Autodesk Fusion 360 part; units mm, degrees
(part 6 of 8)
equation "d149 = FootHeight"
equation "d151 = ( BaseX + TowerFrame + TowerClearance ) + ( ( ( TowerWidth - 2 * ( TowerFrame + TowerClearance ) ) - 11 mm ) - PegSize / 2 - FitClearance )"
equation "d152 = ( BaseY ) + ( ( 11 mm ) - PegSize / 2 - FitClearance )"
equation "d153 = PegSize + 2 * FitClearance"
equation "d154 = PegSize + 2 * FitClearance"
equation "d155 = PegHeight + 0.3 mm"
equation "d157 = FootHeight"
equation "d159 = ( BaseX + TowerFrame + TowerClearance ) + ( ( ( TowerWidth - 2 * ( TowerFrame + TowerClearance ) ) - 11 mm ) - PegSize / 2 - FitClearance )"
equation "d160 = ( BaseY ) + ( ( ( Depth ) - 11 mm ) - PegSize / 2 - FitClearance )"
equation "d161 = PegSize + 2 * FitClearance"
equation "d162 = PegSize + 2 * FitClearance"
equation "d163 = PegHeight + 0.3 mm"
equation "d165 = ( FootHeight ) + PanHeight - DeckThick"
equation "d167 = ( BaseX + TowerFrame + TowerClearance ) + ( Wall + DeckClearance )"
equation "d168 = ( BaseY ) + ( Wall + DeckClearance )"
equation "d169 = ( TowerWidth - 2 * ( TowerFrame + TowerClearance ) ) - 2 * ( Wall + DeckClearance )"
equation "d170 = ( Depth ) - 2 * ( Wall + DeckClearance )"
equation "d171 = DeckThick"
equation "d173 = ( FootHeight ) + PanHeight - DeckThick"
equation "d175 = ( BaseX + TowerFrame + TowerClearance ) + ( ( ( ( TowerWidth - 2 * ( TowerFrame + TowerClearance ) ) - ( 12 * SlotPitch + SlotWidth ) ) / 2 ) + ( 0 * SlotPitch ) )"
equation "d176 = ( BaseY ) + ( Wall + DeckClearance + RimBorder )"
equation "d177 = SlotWidth"
equation "d178 = ( Depth ) - 2 * ( Wall + DeckClearance + RimBorder )"
equation "d179 = DeckThick"
equation "d181 = ( FootHeight ) + PanHeight - DeckThick"
equation "d183 = ( BaseX + TowerFrame + TowerClearance ) + ( ( ( ( TowerWidth - 2 * ( TowerFrame + TowerClearance ) ) - ( 12 * SlotPitch + SlotWidth ) ) / 2 ) + ( 1 * SlotPitch ) )"
equation "d184 = ( BaseY ) + ( Wall + DeckClearance + RimBorder )"
equation "d185 = SlotWidth"
equation "d186 = ( Depth ) - 2 * ( Wall + DeckClearance + RimBorder )"
equation "d187 = DeckThick"
equation "d189 = ( FootHeight ) + PanHeight - DeckThick"
equation "d191 = ( BaseX + TowerFrame + TowerClearance ) + ( ( ( ( TowerWidth - 2 * ( TowerFrame + TowerClearance ) ) - ( 12 * SlotPitch + SlotWidth ) ) / 2 ) + ( 2 * SlotPitch ) )"
equation "d192 = ( BaseY ) + ( Wall + DeckClearance + RimBorder )"
equation "d193 = SlotWidth"
equation "d194 = ( Depth ) - 2 * ( Wall + DeckClearance + RimBorder )"
equation "d195 = DeckThick"
equation "d197 = ( FootHeight ) + PanHeight - DeckThick"
equation "d199 = ( BaseX + TowerFrame + TowerClearance ) + ( ( ( ( TowerWidth - 2 * ( TowerFrame + TowerClearance ) ) - ( 12 * SlotPitch + SlotWidth ) ) / 2 ) + ( 3 * SlotPitch ) )"
equation "d200 = ( BaseY ) + ( Wall + DeckClearance + RimBorder )"
equation "d201 = SlotWidth"
equation "d202 = ( Depth ) - 2 * ( Wall + DeckClearance + RimBorder )"
equation "d203 = DeckThick"
equation "d205 = ( FootHeight ) + PanHeight - DeckThick"
equation "d207 = ( BaseX + TowerFrame + TowerClearance ) + ( ( ( ( TowerWidth - 2 * ( TowerFrame + TowerClearance ) ) - ( 12 * SlotPitch + SlotWidth ) ) / 2 ) + ( 4 * SlotPitch ) )"
equation "d208 = ( BaseY ) + ( Wall + DeckClearance + RimBorder )"
equation "d209 = SlotWidth"
equation "d210 = ( Depth ) - 2 * ( Wall + DeckClearance + RimBorder )"
equation "d211 = DeckThick"
equation "d213 = ( FootHeight ) + PanHeight - DeckThick"
equation "d215 = ( BaseX + TowerFrame + TowerClearance ) + ( ( ( ( TowerWidth - 2 * ( TowerFrame + TowerClearance ) ) - ( 12 * SlotPitch + SlotWidth ) ) / 2 ) + ( 5 * SlotPitch ) )"
equation "d216 = ( BaseY ) + ( Wall + DeckClearance + RimBorder )"
equation "d217 = SlotWidth"
equation "d218 = ( Depth ) - 2 * ( Wall + DeckClearance + RimBorder )"
equation "d219 = DeckThick"
equation "d221 = ( FootHeight ) + PanHeight - DeckThick"
equation "d223 = ( BaseX + TowerFrame + TowerClearance ) + ( ( ( ( TowerWidth - 2 * ( TowerFrame + TowerClearance ) ) - ( 12 * SlotPitch + SlotWidth ) ) / 2 ) + ( 6 * SlotPitch ) )"
equation "d224 = ( BaseY ) + ( Wall + DeckClearance + RimBorder )"
equation "d225 = SlotWidth"
equation "d226 = ( Depth ) - 2 * ( Wall + DeckClearance + RimBorder )"
equation "d227 = DeckThick"
equation "d229 = ( FootHeight ) + PanHeight - DeckThick"
equation "d231 = ( BaseX + TowerFrame + TowerClearance ) + ( ( ( ( TowerWidth - 2 * ( TowerFrame + TowerClearance ) ) - ( 12 * SlotPitch + SlotWidth ) ) / 2 ) + ( 7 * SlotPitch ) )"
equation "d232 = ( BaseY ) + ( Wall + DeckClearance + RimBorder )"
equation "d233 = SlotWidth"
equation "d234 = ( Depth ) - 2 * ( Wall + DeckClearance + RimBorder )"
equation "d235 = DeckThick"
equation "d237 = ( FootHeight ) + PanHeight - DeckThick"
equation "d239 = ( BaseX + TowerFrame + TowerClearance ) + ( ( ( ( TowerWidth - 2 * ( TowerFrame + TowerClearance ) ) - ( 12 * SlotPitch + SlotWidth ) ) / 2 ) + ( 8 * SlotPitch ) )"
equation "d240 = ( BaseY ) + ( Wall + DeckClearance + RimBorder )"
equation "d241 = SlotWidth"
equation "d242 = ( Depth ) - 2 * ( Wall + DeckClearance + RimBorder )"
equation "d243 = DeckThick"
equation "d245 = ( FootHeight ) + PanHeight - DeckThick"
equation "d247 = ( BaseX + TowerFrame + TowerClearance ) + ( ( ( ( TowerWidth - 2 * ( TowerFrame + TowerClearance ) ) - ( 12 * SlotPitch + SlotWidth ) ) / 2 ) + ( 9 * SlotPitch ) )"
equation "d248 = ( BaseY ) + ( Wall + DeckClearance + RimBorder )"
equation "d249 = SlotWidth"
equation "d250 = ( Depth ) - 2 * ( Wall + DeckClearance + RimBorder )"
equation "d251 = DeckThick"
equation "d253 = ( FootHeight ) + PanHeight - DeckThick"
equation "d255 = ( BaseX + TowerFrame + TowerClearance ) + ( ( ( ( TowerWidth - 2 * ( TowerFrame + TowerClearance ) ) - ( 12 * SlotPitch + SlotWidth ) ) / 2 ) + ( 10 * SlotPitch ) )"
equation "d256 = ( BaseY ) + ( Wall + DeckClearance + RimBorder )"
equation "d257 = SlotWidth"
equation "d258 = ( Depth ) - 2 * ( Wall + DeckClearance + RimBorder )"
equation "d259 = DeckThick"
equation "d261 = ( FootHeight ) + PanHeight - DeckThick"
equation "d263 = ( BaseX + TowerFrame + TowerClearance ) + ( ( ( ( TowerWidth - 2 * ( TowerFrame + TowerClearance ) ) - ( 12 * SlotPitch + SlotWidth ) ) / 2 ) + ( 11 * SlotPitch ) )"
equation "d264 = ( BaseY ) + ( Wall + DeckClearance + RimBorder )"
equation "d265 = SlotWidth"
equation "d266 = ( Depth ) - 2 * ( Wall + DeckClearance + RimBorder )"
equation "d267 = DeckThick"
equation "d269 = ( FootHeight ) + PanHeight - DeckThick"
equation "d271 = ( BaseX + TowerFrame + TowerClearance ) + ( ( ( ( TowerWidth - 2 * ( TowerFrame + TowerClearance ) ) - ( 12 * SlotPitch + SlotWidth ) ) / 2 ) + ( 12 * SlotPitch ) )"
equation "d272 = ( BaseY ) + ( Wall + DeckClearance + RimBorder )"
equation "d273 = SlotWidth"
equation "d274 = ( Depth ) - 2 * ( Wall + DeckClearance + RimBorder )"
equation "d275 = DeckThick"
equation "d277 = ( FootHeight ) + PanHeight - DeckThick"
equation "d279 = ( BaseX + TowerFrame + TowerClearance ) + ( ( TowerWidth - 2 * ( TowerFrame + TowerClearance ) ) / 2 - 8 mm )"
equation "d280 = ( BaseY ) + ( ( Depth ) - Wall - DeckClearance - 4 mm )"
equation "d283 = DeckThick"
equation "d287 = ( BaseX + TowerFrame + TowerClearance ) + ( ( 11 mm ) - FootSize / 2 )"
equation "d288 = ( BaseY ) + ( ( 11 mm ) - FootSize / 2 )"
equation "d289 = FootSize"
equation "d290 = FootSize"
equation "d291 = FootHeight"
equation "d293 = FootHeight"
equation "d295 = ( BaseX + TowerFrame + TowerClearance ) + ( ( 11 mm ) - PegSize / 2 )"
equation "d296 = ( BaseY ) + ( ( 11 mm ) - PegSize / 2 )"
equation "d297 = PegSize"
equation "d298 = PegSize"
equation "d299 = PegHeight"
equation "d303 = ( BaseX + TowerFrame + TowerClearance ) + ( ( 11 mm ) - FootSize / 2 )"
equation "d304 = ( BaseY ) + ( ( ( Depth ) - 11 mm ) - FootSize / 2 )"
equation "d305 = FootSize"
equation "d306 = FootSize"
equation "d307 = FootHeight"
equation "d309 = FootHeight"
equation "d311 = ( BaseX + TowerFrame + TowerClearance ) + ( ( 11 mm ) - PegSize / 2 )"
equation "d312 = ( BaseY ) + ( ( ( Depth ) - 11 mm ) - PegSize / 2 )"
equation "d313 = PegSize"
equation "d314 = PegSize"
equation "d315 = PegHeight"
equation "d319 = ( BaseX + TowerFrame + TowerClearance ) + ( ( ( TowerWidth - 2 * ( TowerFrame + TowerClearance ) ) - 11 mm ) - FootSize / 2 )"
equation "d320 = ( BaseY ) + ( ( 11 mm ) - FootSize / 2 )"
equation "d321 = FootSize"
equation "d322 = FootSize"
equation "d323 = FootHeight"
equation "d325 = FootHeight"
equation "d327 = ( BaseX + TowerFrame + TowerClearance ) + ( ( ( TowerWidth - 2 * ( TowerFrame + TowerClearance ) ) - 11 mm ) - PegSize / 2 )"
equation "d328 = ( BaseY ) + ( ( 11 mm ) - PegSize / 2 )"
equation "d329 = PegSize"
equation "d330 = PegSize"
equation "d331 = PegHeight"
equation "d335 = ( BaseX + TowerFrame + TowerClearance ) + ( ( ( TowerWidth - 2 * ( TowerFrame + TowerClearance ) ) - 11 mm ) - FootSize / 2 )"
equation "d336 = ( BaseY ) + ( ( ( Depth ) - 11 mm ) - FootSize / 2 )"
equation "d337 = FootSize"
equation "d338 = FootSize"
equation "d339 = FootHeight"
equation "d341 = FootHeight"
equation "d343 = ( BaseX + TowerFrame + TowerClearance ) + ( ( ( TowerWidth - 2 * ( TowerFrame + TowerClearance ) ) - 11 mm ) - PegSize / 2 )"
equation "d344 = ( BaseY ) + ( ( ( Depth ) - 11 mm ) - PegSize / 2 )"
equation "d345 = PegSize"
equation "d346 = PegSize"
equation "d347 = PegHeight"
equation "d349 = FootHeight"
equation "d351 = ( BaseX + TowerWidth + ModuleGap ) + ( 0 mm )"
equation "d352 = ( BaseY ) + ( 0 mm )"
equation "d353 = LeftRun - TowerWidth - ModuleGap"
equation "d354 = Depth"
equation "d355 = PanHeight"
equation "d359 = ( BaseX + TowerWidth + ModuleGap ) + ( Wall )"
equation "d361 = -( -( ( FootHeight ) + FloorMin + DrainExtension * tan(DrainSlope) + ( ( Depth ) - ( Wall ) ) * tan(DrainSlope) ) )"
equation "d362 = ( ( BaseY ) + ( Wall ) )"
equation "d363 = -( -( ( FootHeight ) + FloorMin + DrainExtension * tan(DrainSlope) + ( ( Depth ) - ( ( Depth ) - Wall ) ) * tan(DrainSlope) ) )"
equation "d364 = ( ( BaseY ) + ( ( Depth ) - Wall ) )"
equation "d365 = -( -( ( FootHeight ) + PanHeight + 1 mm ) )"
equation "d366 = ( LeftRun - TowerWidth - ModuleGap ) - 2 * Wall"
equation "d368 = ( BaseX + TowerWidth + ModuleGap ) + ( ( ( LeftRun - TowerWidth - ModuleGap ) / 2 ) - DrainWidth / 2 - Wall )"
equation "d370 = -( -( FootHeight ) )"
equation "d371 = ( ( BaseY ) + ( ( Depth ) - Wall ) )"
equation "d372 = ( ( BaseY ) + ( ( Depth ) + DrainExtension ) )"
equation "d373 = -( -( ( FootHeight ) + FloorMin + DrainExtension * tan(DrainSlope) + ( ( Depth ) - ( ( Depth ) + DrainExtension ) ) * tan(DrainSlope) ) )"
equation "d374 = -( -( ( FootHeight ) + FloorMin + DrainExtension * tan(DrainSlope) + ( ( Depth ) - ( ( Depth ) - Wall ) ) * tan(DrainSlope) ) )"
equation "d375 = DrainWidth + 2 * Wall"
equation "d377 = ( BaseX + TowerWidth + ModuleGap ) + ( ( ( LeftRun - TowerWidth - ModuleGap ) / 2 ) - DrainWidth / 2 - Wall )"
equation "d379 = -( -( FootHeight ) )"
equation "d380 = ( ( BaseY ) + ( ( Depth ) - Wall ) )"
equation "d381 = ( ( BaseY ) + ( ( Depth ) + DrainExtension ) )"
equation "d382 = -( -( ( ( FootHeight ) + FloorMin + DrainExtension * tan(DrainSlope) + ( ( Depth ) - ( ( Depth ) + DrainExtension ) ) * tan(DrainSlope) ) + ( 6 mm ) ) )"
equation "d383 = -( -( ( ( FootHeight ) + FloorMin + DrainExtension * tan(DrainSlope) + ( ( Depth ) - ( ( Depth ) - Wall ) ) * tan(DrainSlope) ) + ( 6 mm ) ) )"
equation "d384 = Wall"
equation "d386 = ( BaseX + TowerWidth + ModuleGap ) + ( ( ( LeftRun - TowerWidth - ModuleGap ) / 2 ) + DrainWidth / 2 )"
equation "d388 = -( -( FootHeight ) )"
equation "d389 = ( ( BaseY ) + ( ( Depth ) - Wall ) )"
equation "d390 = ( ( BaseY ) + ( ( Depth ) + DrainExtension ) )"
equation "d391 = -( -( ( ( FootHeight ) + FloorMin + DrainExtension * tan(DrainSlope) + ( ( Depth ) - ( ( Depth ) + DrainExtension ) ) * tan(DrainSlope) ) + ( 6 mm ) ) )"
equation "d392 = -( -( ( ( FootHeight ) + FloorMin + DrainExtension * tan(DrainSlope) + ( ( Depth ) - ( ( Depth ) - Wall ) ) * tan(DrainSlope) ) + ( 6 mm ) ) )"
equation "d393 = Wall"
equation "d395 = ( BaseX + TowerWidth + ModuleGap ) + ( ( ( LeftRun - TowerWidth - ModuleGap ) / 2 ) - DrainWidth / 2 )"
equation "d397 = -( -( ( FootHeight ) + FloorMin + DrainExtension * tan(DrainSlope) + ( ( Depth ) - ( ( Depth ) - Wall ) ) * tan(DrainSlope) ) )"
equation "d398 = ( ( BaseY ) + ( ( Depth ) - Wall ) )"
equation "d399 = -( -( ( FootHeight ) + FloorMin + DrainExtension * tan(DrainSlope) + ( ( Depth ) - ( ( Depth ) + DrainExtension ) ) * tan(DrainSlope) ) )"
equation "d400 = ( ( BaseY ) + ( ( Depth ) + DrainExtension ) )"
equation "d401 = -( -( ( FootHeight ) + PanHeight + 1 mm ) )"
equation "d402 = DrainWidth"
equation "d404 = FootHeight"
equation "d406 = ( BaseX + TowerWidth + ModuleGap ) + ( Wall )"
equation "d407 = ( BaseY ) + ( Wall )"
equation "d410 = PanHeight - DeckThick"
equation "d412 = FootHeight"
equation "d414 = ( BaseX + TowerWidth + ModuleGap ) + ( Wall )"
equation "d415 = ( BaseY ) + ( ( Depth ) - Wall - 12 mm )"
equation "d418 = PanHeight - DeckThick"
equation "d420 = FootHeight"
equation "d422 = ( BaseX + TowerWidth + ModuleGap ) + ( ( LeftRun - TowerWidth - ModuleGap ) - Wall - 12 mm )"
equation "d423 = ( BaseY ) + ( Wall )"
equation "d426 = PanHeight - DeckThick"
equation "d428 = FootHeight"
equation "d430 = ( BaseX + TowerWidth + ModuleGap ) + ( ( LeftRun - TowerWidth - ModuleGap ) - Wall - 12 mm )"
equation "d431 = ( BaseY ) + ( ( Depth ) - Wall - 12 mm )"
equation "d434 = PanHeight - DeckThick"
equation "d436 = ( BaseX + TowerWidth + ModuleGap ) + ( ( ( LeftRun - TowerWidth - ModuleGap ) / 2 ) - DrainWidth / 2 - Wall )"
equation "d438 = -( -( ( FootHeight ) - ( 0.2 mm ) ) )"
equation "d439 = ( ( BaseY ) + ( ( Depth ) + DrainExtension - 2 mm ) )"
equation "d440 = ( ( BaseY ) + ( ( ( Depth ) + DrainExtension - 2 mm ) + ( 1 mm ) ) )"
equation "d441 = -( -( ( FootHeight ) + ( 0.6 mm ) ) )"
equation "d442 = DrainWidth + 2 * Wall"
equation "d444 = FootHeight"
equation "d446 = ( BaseX + TowerWidth + ModuleGap ) + ( ( 11 mm ) - PegSize / 2 - FitClearance )"
equation "d447 = ( BaseY ) + ( ( 11 mm ) - PegSize / 2 - FitClearance )"
equation "d448 = PegSize + 2 * FitClearance"
equation "d449 = PegSize + 2 * FitClearance"
equation "d450 = PegHeight + 0.3 mm"
equation "d452 = FootHeight"
equation "d454 = ( BaseX + TowerWidth + ModuleGap ) + ( ( 11 mm ) - PegSize / 2 - FitClearance )"
equation "d455 = ( BaseY ) + ( ( ( Depth ) - 11 mm ) - PegSize / 2 - FitClearance )"
equation "d456 = PegSize + 2 * FitClearance"
equation "d457 = PegSize + 2 * FitClearance"
equation "d458 = PegHeight + 0.3 mm"
equation "d460 = FootHeight"
equation "d462 = ( BaseX + TowerWidth + ModuleGap ) + ( ( ( LeftRun - TowerWidth - ModuleGap ) - 11 mm ) - PegSize / 2 - FitClearance )"
equation "d463 = ( BaseY ) + ( ( 11 mm ) - PegSize / 2 - FitClearance )"
equation "d464 = PegSize + 2 * FitClearance"
equation "d465 = PegSize + 2 * FitClearance"
equation "d466 = PegHeight + 0.3 mm"
equation "d468 = FootHeight"
equation "d470 = ( BaseX + TowerWidth + ModuleGap ) + ( ( ( LeftRun - TowerWidth - ModuleGap ) - 11 mm ) - PegSize / 2 - FitClearance )"
equation "d471 = ( BaseY ) + ( ( ( Depth ) - 11 mm ) - PegSize / 2 - FitClearance )"
equation "d472 = PegSize + 2 * FitClearance"
equation "d473 = PegSize + 2 * FitClearance"
equation "d474 = PegHeight + 0.3 mm"
equation "d476 = ( FootHeight ) + PanHeight - DeckThick"
equation "d478 = ( BaseX + TowerWidth + ModuleGap ) + ( Wall + DeckClearance )"
equation "d479 = ( BaseY ) + ( Wall + DeckClearance )"
equation "d480 = ( LeftRun - TowerWidth - ModuleGap ) - 2 * ( Wall + DeckClearance )"
equation "d481 = ( Depth ) - 2 * ( Wall + DeckClearance )"
equation "d482 = DeckThick"
equation "d484 = ( FootHeight ) + PanHeight - DeckThick"
equation "d486 = ( BaseX + TowerWidth + ModuleGap ) + ( ( ( ( LeftRun - TowerWidth - ModuleGap ) - ( 16 * SlotPitch + SlotWidth ) ) / 2 ) + ( 0 * SlotPitch ) )"
equation "d487 = ( BaseY ) + ( Wall + DeckClearance + RimBorder )"
equation "d488 = SlotWidth"
equation "d489 = ( Depth ) - 2 * ( Wall + DeckClearance + RimBorder )"
equation "d490 = DeckThick"
equation "d492 = ( FootHeight ) + PanHeight - DeckThick"
equation "d494 = ( BaseX + TowerWidth + ModuleGap ) + ( ( ( ( LeftRun - TowerWidth - ModuleGap ) - ( 16 * SlotPitch + SlotWidth ) ) / 2 ) + ( 1 * SlotPitch ) )"
equation "d495 = ( BaseY ) + ( Wall + DeckClearance + RimBorder )"
equation "d496 = SlotWidth"
equation "d497 = ( Depth ) - 2 * ( Wall + DeckClearance + RimBorder )"
equation "d498 = DeckThick"
equation "d500 = ( FootHeight ) + PanHeight - DeckThick"
equation "d502 = ( BaseX + TowerWidth + ModuleGap ) + ( ( ( ( LeftRun - TowerWidth - ModuleGap ) - ( 16 * SlotPitch + SlotWidth ) ) / 2 ) + ( 2 * SlotPitch ) )"
equation "d503 = ( BaseY ) + ( Wall + DeckClearance + RimBorder )"
equation "d504 = SlotWidth"
equation "d505 = ( Depth ) - 2 * ( Wall + DeckClearance + RimBorder )"
equation "d506 = DeckThick"
equation "d508 = ( FootHeight ) + PanHeight - DeckThick"
equation "d510 = ( BaseX + TowerWidth + ModuleGap ) + ( ( ( ( LeftRun - TowerWidth - ModuleGap ) - ( 16 * SlotPitch + SlotWidth ) ) / 2 ) + ( 3 * SlotPitch ) )"
equation "d511 = ( BaseY ) + ( Wall + DeckClearance + RimBorder )"
equation "d512 = SlotWidth"
equation "d513 = ( Depth ) - 2 * ( Wall + DeckClearance + RimBorder )"
equation "d514 = DeckThick"
equation "d516 = ( FootHeight ) + PanHeight - DeckThick"
equation "d518 = ( BaseX + TowerWidth + ModuleGap ) + ( ( ( ( LeftRun - TowerWidth - ModuleGap ) - ( 16 * SlotPitch + SlotWidth ) ) / 2 ) + ( 4 * SlotPitch ) )"
equation "d519 = ( BaseY ) + ( Wall + DeckClearance + RimBorder )"
equation "d520 = SlotWidth"
equation "d521 = ( Depth ) - 2 * ( Wall + DeckClearance + RimBorder )"
equation "d522 = DeckThick"
equation "d524 = ( FootHeight ) + PanHeight - DeckThick"
equation "d526 = ( BaseX + TowerWidth + ModuleGap ) + ( ( ( ( LeftRun - TowerWidth - ModuleGap ) - ( 16 * SlotPitch + SlotWidth ) ) / 2 ) + ( 5 * SlotPitch ) )"
equation "d527 = ( BaseY ) + ( Wall + DeckClearance + RimBorder )"
equation "d528 = SlotWidth"
equation "d529 = ( Depth ) - 2 * ( Wall + DeckClearance + RimBorder )"
equation "d530 = DeckThick"
equation "d532 = ( FootHeight ) + PanHeight - DeckThick"
equation "d534 = ( BaseX + TowerWidth + ModuleGap ) + ( ( ( ( LeftRun - TowerWidth - ModuleGap ) - ( 16 * SlotPitch + SlotWidth ) ) / 2 ) + ( 6 * SlotPitch ) )"
equation "d535 = ( BaseY ) + ( Wall + DeckClearance + RimBorder )"
equation "d536 = SlotWidth"
equation "d537 = ( Depth ) - 2 * ( Wall + DeckClearance + RimBorder )"
equation "d538 = DeckThick"
equation "d540 = ( FootHeight ) + PanHeight - DeckThick"
equation "d542 = ( BaseX + TowerWidth + ModuleGap ) + ( ( ( ( LeftRun - TowerWidth - ModuleGap ) - ( 16 * SlotPitch + SlotWidth ) ) / 2 ) + ( 7 * SlotPitch ) )"
equation "d543 = ( BaseY ) + ( Wall + DeckClearance + RimBorder )"
equation "d544 = SlotWidth"
equation "d545 = ( Depth ) - 2 * ( Wall + DeckClearance + RimBorder )"
equation "d546 = DeckThick"
equation "d548 = ( FootHeight ) + PanHeight - DeckThick"
equation "d550 = ( BaseX + TowerWidth + ModuleGap ) + ( ( ( ( LeftRun - TowerWidth - ModuleGap ) - ( 16 * SlotPitch + SlotWidth ) ) / 2 ) + ( 8 * SlotPitch ) )"
equation "d551 = ( BaseY ) + ( Wall + DeckClearance + RimBorder )"
equation "d552 = SlotWidth"
equation "d553 = ( Depth ) - 2 * ( Wall + DeckClearance + RimBorder )"
equation "d554 = DeckThick"
equation "d556 = ( FootHeight ) + PanHeight - DeckThick"
equation "d558 = ( BaseX + TowerWidth + ModuleGap ) + ( ( ( ( LeftRun - TowerWidth - ModuleGap ) - ( 16 * SlotPitch + SlotWidth ) ) / 2 ) + ( 9 * SlotPitch ) )"
equation "d559 = ( BaseY ) + ( Wall + DeckClearance + RimBorder )"
equation "d560 = SlotWidth"
equation "d561 = ( Depth ) - 2 * ( Wall + DeckClearance + RimBorder )"
equation "d562 = DeckThick"
equation "d564 = ( FootHeight ) + PanHeight - DeckThick"
equation "d566 = ( BaseX + TowerWidth + ModuleGap ) + ( ( ( ( LeftRun - TowerWidth - ModuleGap ) - ( 16 * SlotPitch + SlotWidth ) ) / 2 ) + ( 10 * SlotPitch ) )"
equation "d567 = ( BaseY ) + ( Wall + DeckClearance + RimBorder )"
equation "d568 = SlotWidth"
equation "d569 = ( Depth ) - 2 * ( Wall + DeckClearance + RimBorder )"
equation "d570 = DeckThick"
equation "d572 = ( FootHeight ) + PanHeight - DeckThick"
equation "d574 = ( BaseX + TowerWidth + ModuleGap ) + ( ( ( ( LeftRun - TowerWidth - ModuleGap ) - ( 16 * SlotPitch + SlotWidth ) ) / 2 ) + ( 11 * SlotPitch ) )"
equation "d575 = ( BaseY ) + ( Wall + DeckClearance + RimBorder )"
equation "d576 = SlotWidth"
equation "d577 = ( Depth ) - 2 * ( Wall + DeckClearance + RimBorder )"
equation "d578 = DeckThick"
equation "d580 = ( FootHeight ) + PanHeight - DeckThick"
equation "d582 = ( BaseX + TowerWidth + ModuleGap ) + ( ( ( ( LeftRun - TowerWidth - ModuleGap ) - ( 16 * SlotPitch + SlotWidth ) ) / 2 ) + ( 12 * SlotPitch ) )"
equation "d583 = ( BaseY ) + ( Wall + DeckClearance + RimBorder )"
equation "d584 = SlotWidth"
equation "d585 = ( Depth ) - 2 * ( Wall + DeckClearance + RimBorder )"
equation "d586 = DeckThick"
equation "d588 = ( FootHeight ) + PanHeight - DeckThick"
equation "d590 = ( BaseX + TowerWidth + ModuleGap ) + ( ( ( ( LeftRun - TowerWidth - ModuleGap ) - ( 16 * SlotPitch + SlotWidth ) ) / 2 ) + ( 13 * SlotPitch ) )"
equation "d591 = ( BaseY ) + ( Wall + DeckClearance + RimBorder )"
equation "d592 = SlotWidth"
equation "d593 = ( Depth ) - 2 * ( Wall + DeckClearance + RimBorder )"
equation "d594 = DeckThick"
equation "d596 = ( FootHeight ) + PanHeight - DeckThick"
equation "d598 = ( BaseX + TowerWidth + ModuleGap ) + ( ( ( ( LeftRun - TowerWidth - ModuleGap ) - ( 16 * SlotPitch + SlotWidth ) ) / 2 ) + ( 14 * SlotPitch ) )"
equation "d599 = ( BaseY ) + ( Wall + DeckClearance + RimBorder )"
equation "d600 = SlotWidth"
equation "d601 = ( Depth ) - 2 * ( Wall + DeckClearance + RimBorder )"
equation "d602 = DeckThick"
equation "d604 = ( FootHeight ) + PanHeight - DeckThick"
equation "d606 = ( BaseX + TowerWidth + ModuleGap ) + ( ( ( ( LeftRun - TowerWidth - ModuleGap ) - ( 16 * SlotPitch + SlotWidth ) ) / 2 ) + ( 15 * SlotPitch ) )"
equation "d607 = ( BaseY ) + ( Wall + DeckClearance + RimBorder )"
equation "d608 = SlotWidth"
equation "d609 = ( Depth ) - 2 * ( Wall + DeckClearance + RimBorder )"
equation "d610 = DeckThick"
equation "d612 = ( FootHeight ) + PanHeight - DeckThick"
equation "d614 = ( BaseX + TowerWidth + ModuleGap ) + ( ( ( ( LeftRun - TowerWidth - ModuleGap ) - ( 16 * SlotPitch + SlotWidth ) ) / 2 ) + ( 16 * SlotPitch ) )"
equation "d615 = ( BaseY ) + ( Wall + DeckClearance + RimBorder )"
equation "d616 = SlotWidth"
equation "d617 = ( Depth ) - 2 * ( Wall + DeckClearance + RimBorder )"
equation "d618 = DeckThick"
equation "d620 = ( FootHeight ) + PanHeight - DeckThick"
equation "d622 = ( BaseX + TowerWidth + ModuleGap ) + ( ( LeftRun - TowerWidth - ModuleGap ) / 2 - 8 mm )"
equation "d623 = ( BaseY ) + ( ( Depth ) - Wall - DeckClearance - 4 mm )"
equation "d626 = DeckThick"
equation "d630 = ( BaseX + TowerWidth + ModuleGap ) + ( ( 11 mm ) - FootSize / 2 )"
equation "d631 = ( BaseY ) + ( ( 11 mm ) - FootSize / 2 )"
equation "d632 = FootSize"
equation "d633 = FootSize"
equation "d634 = FootHeight"
equation "d636 = FootHeight"
equation "d638 = ( BaseX + TowerWidth + ModuleGap ) + ( ( 11 mm ) - PegSize / 2 )"
equation "d639 = ( BaseY ) + ( ( 11 mm ) - PegSize / 2 )"
equation "d640 = PegSize"
equation "d641 = PegSize"
equation "d642 = PegHeight"
equation "d646 = ( BaseX + TowerWidth + ModuleGap ) + ( ( 11 mm ) - FootSize / 2 )"
equation "d647 = ( BaseY ) + ( ( ( Depth ) - 11 mm ) - FootSize / 2 )"
equation "d648 = FootSize"
equation "d649 = FootSize"
equation "d650 = FootHeight"
equation "d652 = FootHeight"
equation "d654 = ( BaseX + TowerWidth + ModuleGap ) + ( ( 11 mm ) - PegSize / 2 )"
equation "d655 = ( BaseY ) + ( ( ( Depth ) - 11 mm ) - PegSize / 2 )"
equation "d656 = PegSize"
equation "d657 = PegSize"
equation "d658 = PegHeight"
equation "d662 = ( BaseX + TowerWidth + ModuleGap ) + ( ( ( LeftRun - TowerWidth - ModuleGap ) - 11 mm ) - FootSize / 2 )"
equation "d663 = ( BaseY ) + ( ( 11 mm ) - FootSize / 2 )"
equation "d664 = FootSize"
equation "d665 = FootSize"
equation "d666 = FootHeight"
equation "d668 = FootHeight"
equation "d670 = ( BaseX + TowerWidth + ModuleGap ) + ( ( ( LeftRun - TowerWidth - ModuleGap ) - 11 mm ) - PegSize / 2 )"
equation "d671 = ( BaseY ) + ( ( 11 mm ) - PegSize / 2 )"
equation "d672 = PegSize"
equation "d673 = PegSize"
equation "d674 = PegHeight"
equation "d678 = ( BaseX + TowerWidth + ModuleGap ) + ( ( ( LeftRun - TowerWidth - ModuleGap ) - 11 mm ) - FootSize / 2 )"
equation "d679 = ( BaseY ) + ( ( ( Depth ) - 11 mm ) - FootSize / 2 )"
equation "d680 = FootSize"
equation "d681 = FootSize"
equation "d682 = FootHeight"
equation "d684 = FootHeight"
equation "d686 = ( BaseX + TowerWidth + ModuleGap ) + ( ( ( LeftRun - TowerWidth - ModuleGap ) - 11 mm ) - PegSize / 2 )"
equation "d687 = ( BaseY ) + ( ( ( Depth ) - 11 mm ) - PegSize / 2 )"
equation "d688 = PegSize"
equation "d689 = PegSize"
equation "d690 = PegHeight"
equation "d692 = FootHeight"
equation "d694 = ( BaseX + LeftRun + FaucetGap ) + ( 0 mm )"
equation "d695 = ( BaseY ) + ( 0 mm )"
equation "d696 = ( RightRun - ModuleGap ) / 2"
equation "d697 = Depth"
equation "d698 = PanHeight"
equation "d702 = ( BaseX + LeftRun + FaucetGap ) + ( Wall )"
equation "d704 = -( -( ( FootHeight ) + FloorMin + DrainExtension * tan(DrainSlope) + ( ( Depth ) - ( Wall ) ) * tan(DrainSlope) ) )"
equation "d705 = ( ( BaseY ) + ( Wall ) )"
equation "d706 = -( -( ( FootHeight ) + FloorMin + DrainExtension * tan(DrainSlope) + ( ( Depth ) - ( ( Depth ) - Wall ) ) * tan(DrainSlope) ) )"
equation "d707 = ( ( BaseY ) + ( ( Depth ) - Wall ) )"
equation "d708 = -( -( ( FootHeight ) + PanHeight + 1 mm ) )"
equation "d709 = ( ( RightRun - ModuleGap ) / 2 ) - 2 * Wall"
equation "d711 = ( BaseX + LeftRun + FaucetGap ) + ( ( ( RightRun - ModuleGap ) / 4 ) - DrainWidth / 2 - Wall )"
equation "d713 = -( -( FootHeight ) )"
equation "d714 = ( ( BaseY ) + ( ( Depth ) - Wall ) )"
equation "d715 = ( ( BaseY ) + ( ( Depth ) + DrainExtension ) )"
equation "d716 = -( -( ( FootHeight ) + FloorMin + DrainExtension * tan(DrainSlope) + ( ( Depth ) - ( ( Depth ) + DrainExtension ) ) * tan(DrainSlope) ) )"
equation "d717 = -( -( ( FootHeight ) + FloorMin + DrainExtension * tan(DrainSlope) + ( ( Depth ) - ( ( Depth ) - Wall ) ) * tan(DrainSlope) ) )"
equation "d718 = DrainWidth + 2 * Wall"
equation "d720 = ( BaseX + LeftRun + FaucetGap ) + ( ( ( RightRun - ModuleGap ) / 4 ) - DrainWidth / 2 - Wall )"
equation "d722 = -( -( FootHeight ) )"
equation "d723 = ( ( BaseY ) + ( ( Depth ) - Wall ) )"
equation "d724 = ( ( BaseY ) + ( ( Depth ) + DrainExtension ) )"
equation "d725 = -( -( ( ( FootHeight ) + FloorMin + DrainExtension * tan(DrainSlope) + ( ( Depth ) - ( ( Depth ) + DrainExtension ) ) * tan(DrainSlope) ) + ( 6 mm ) ) )"
equation "d726 = -( -( ( ( FootHeight ) + FloorMin + DrainExtension * tan(DrainSlope) + ( ( Depth ) - ( ( Depth ) - Wall ) ) * tan(DrainSlope) ) + ( 6 mm ) ) )"
equation "d727 = Wall"
equation "d729 = ( BaseX + LeftRun + FaucetGap ) + ( ( ( RightRun - ModuleGap ) / 4 ) + DrainWidth / 2 )"
equation "d731 = -( -( FootHeight ) )"
equation "d732 = ( ( BaseY ) + ( ( Depth ) - Wall ) )"
equation "d733 = ( ( BaseY ) + ( ( Depth ) + DrainExtension ) )"
equation "d734 = -( -( ( ( FootHeight ) + FloorMin + DrainExtension * tan(DrainSlope) + ( ( Depth ) - ( ( Depth ) + DrainExtension ) ) * tan(DrainSlope) ) + ( 6 mm ) ) )"
equation "d735 = -( -( ( ( FootHeight ) + FloorMin + DrainExtension * tan(DrainSlope) + ( ( Depth ) - ( ( Depth ) - Wall ) ) * tan(DrainSlope) ) + ( 6 mm ) ) )"
equation "d736 = Wall"
equation "d738 = ( BaseX + LeftRun + FaucetGap ) + ( ( ( RightRun - ModuleGap ) / 4 ) - DrainWidth / 2 )"
equation "d740 = -( -( ( FootHeight ) + FloorMin + DrainExtension * tan(DrainSlope) + ( ( Depth ) - ( ( Depth ) - Wall ) ) * tan(DrainSlope) ) )"
equation "d741 = ( ( BaseY ) + ( ( Depth ) - Wall ) )"
equation "d742 = -( -( ( FootHeight ) + FloorMin + DrainExtension * tan(DrainSlope) + ( ( Depth ) - ( ( Depth ) + DrainExtension ) ) * tan(DrainSlope) ) )"
equation "d743 = ( ( BaseY ) + ( ( Depth ) + DrainExtension ) )"
equation "d744 = -( -( ( FootHeight ) + PanHeight + 1 mm ) )"
equation "d745 = DrainWidth"
equation "d747 = FootHeight"
equation "d749 = ( BaseX + LeftRun + FaucetGap ) + ( Wall )"
equation "d750 = ( BaseY ) + ( Wall )"
equation "d753 = PanHeight - DeckThick"
equation "d755 = FootHeight"
equation "d757 = ( BaseX + LeftRun + FaucetGap ) + ( Wall )"
equation "d758 = ( BaseY ) + ( ( Depth ) - Wall - 12 mm )"
equation "d761 = PanHeight - DeckThick"
equation "d763 = FootHeight"
equation "d765 = ( BaseX + LeftRun + FaucetGap ) + ( ( ( RightRun - ModuleGap ) / 2 ) - Wall - 12 mm )"
equation "d766 = ( BaseY ) + ( Wall )"
equation "d769 = PanHeight - DeckThick"
equation "d771 = FootHeight"
equation "d773 = ( BaseX + LeftRun + FaucetGap ) + ( ( ( RightRun - ModuleGap ) / 2 ) - Wall - 12 mm )"
equation "d774 = ( BaseY ) + ( ( Depth ) - Wall - 12 mm )"
equation "d777 = PanHeight - DeckThick"
equation "d779 = ( BaseX + LeftRun + FaucetGap ) + ( ( ( RightRun - ModuleGap ) / 4 ) - DrainWidth / 2 - Wall )"
equation "d781 = -( -( ( FootHeight ) - ( 0.2 mm ) ) )"
equation "d782 = ( ( BaseY ) + ( ( Depth ) + DrainExtension - 2 mm ) )"
equation "d783 = ( ( BaseY ) + ( ( ( Depth ) + DrainExtension - 2 mm ) + ( 1 mm ) ) )"
equation "d784 = -( -( ( FootHeight ) + ( 0.6 mm ) ) )"
equation "d785 = DrainWidth + 2 * Wall"
equation "d787 = FootHeight"
equation "d789 = ( BaseX + LeftRun + FaucetGap ) + ( ( 11 mm ) - PegSize / 2 - FitClearance )"
equation "d790 = ( BaseY ) + ( ( 11 mm ) - PegSize / 2 - FitClearance )"
equation "d791 = PegSize + 2 * FitClearance"
equation "d792 = PegSize + 2 * FitClearance"
equation "d793 = PegHeight + 0.3 mm"
equation "d795 = FootHeight"
equation "d797 = ( BaseX + LeftRun + FaucetGap ) + ( ( 11 mm ) - PegSize / 2 - FitClearance )"
equation "d798 = ( BaseY ) + ( ( ( Depth ) - 11 mm ) - PegSize / 2 - FitClearance )"
equation "d799 = PegSize + 2 * FitClearance"
equation "d800 = PegSize + 2 * FitClearance"
equation "d801 = PegHeight + 0.3 mm"
equation "d803 = FootHeight"
equation "d805 = ( BaseX + LeftRun + FaucetGap ) + ( ( ( ( RightRun - ModuleGap ) / 2 ) - 11 mm ) - PegSize / 2 - FitClearance )"
equation "d806 = ( BaseY ) + ( ( 11 mm ) - PegSize / 2 - FitClearance )"
equation "d807 = PegSize + 2 * FitClearance"
equation "d808 = PegSize + 2 * FitClearance"
equation "d809 = PegHeight + 0.3 mm"
equation "d811 = FootHeight"
equation "d813 = ( BaseX + LeftRun + FaucetGap ) + ( ( ( ( RightRun - ModuleGap ) / 2 ) - 11 mm ) - PegSize / 2 - FitClearance )"
equation "d814 = ( BaseY ) + ( ( ( Depth ) - 11 mm ) - PegSize / 2 - FitClearance )"
equation "d815 = PegSize + 2 * FitClearance"
equation "d816 = PegSize + 2 * FitClearance"
equation "d817 = PegHeight + 0.3 mm"
equation "d819 = ( FootHeight ) + PanHeight - DeckThick"
equation "d821 = ( BaseX + LeftRun + FaucetGap ) + ( Wall + DeckClearance )"
equation "d822 = ( BaseY ) + ( Wall + DeckClearance )"
equation "d823 = ( ( RightRun - ModuleGap ) / 2 ) - 2 * ( Wall + DeckClearance )"
equation "d824 = ( Depth ) - 2 * ( Wall + DeckClearance )"
equation "d825 = DeckThick"
equation "d827 = ( FootHeight ) + PanHeight - DeckThick"
equation "d829 = ( BaseX + LeftRun + FaucetGap ) + ( ( ( ( ( RightRun - ModuleGap ) / 2 ) - ( 10 * SlotPitch + SlotWidth ) ) / 2 ) + ( 0 * SlotPitch ) )"
equation "d830 = ( BaseY ) + ( Wall + DeckClearance + RimBorder )"
equation "d831 = SlotWidth"
equation "d832 = ( Depth ) - 2 * ( Wall + DeckClearance + RimBorder )"
equation "d833 = DeckThick"
equation "d835 = ( FootHeight ) + PanHeight - DeckThick"
equation "d837 = ( BaseX + LeftRun + FaucetGap ) + ( ( ( ( ( RightRun - ModuleGap ) / 2 ) - ( 10 * SlotPitch + SlotWidth ) ) / 2 ) + ( 1 * SlotPitch ) )"
equation "d838 = ( BaseY ) + ( Wall + DeckClearance + RimBorder )"
equation "d839 = SlotWidth"
equation "d840 = ( Depth ) - 2 * ( Wall + DeckClearance + RimBorder )"
equation "d841 = DeckThick"
equation "d843 = ( FootHeight ) + PanHeight - DeckThick"
equation "d845 = ( BaseX + LeftRun + FaucetGap ) + ( ( ( ( ( RightRun - ModuleGap ) / 2 ) - ( 10 * SlotPitch + SlotWidth ) ) / 2 ) + ( 2 * SlotPitch ) )"
equation "d846 = ( BaseY ) + ( Wall + DeckClearance + RimBorder )"
equation "d847 = SlotWidth"
equation "d848 = ( Depth ) - 2 * ( Wall + DeckClearance + RimBorder )"
equation "d849 = DeckThick"
equation "d851 = ( FootHeight ) + PanHeight - DeckThick"
equation "d853 = ( BaseX + LeftRun + FaucetGap ) + ( ( ( ( ( RightRun - ModuleGap ) / 2 ) - ( 10 * SlotPitch + SlotWidth ) ) / 2 ) + ( 3 * SlotPitch ) )"
equation "d854 = ( BaseY ) + ( Wall + DeckClearance + RimBorder )"
equation "d855 = SlotWidth"
equation "d856 = ( Depth ) - 2 * ( Wall + DeckClearance + RimBorder )"
equation "d857 = DeckThick"
equation "d859 = ( FootHeight ) + PanHeight - DeckThick"
equation "d861 = ( BaseX + LeftRun + FaucetGap ) + ( ( ( ( ( RightRun - ModuleGap ) / 2 ) - ( 10 * SlotPitch + SlotWidth ) ) / 2 ) + ( 4 * SlotPitch ) )"
equation "d862 = ( BaseY ) + ( Wall + DeckClearance + RimBorder )"
equation "d863 = SlotWidth"
equation "d864 = ( Depth ) - 2 * ( Wall + DeckClearance + RimBorder )"
equation "d865 = DeckThick"
equation "d867 = ( FootHeight ) + PanHeight - DeckThick"
equation "d869 = ( BaseX + LeftRun + FaucetGap ) + ( ( ( ( ( RightRun - ModuleGap ) / 2 ) - ( 10 * SlotPitch + SlotWidth ) ) / 2 ) + ( 5 * SlotPitch ) )"
equation "d870 = ( BaseY ) + ( Wall + DeckClearance + RimBorder )"
equation "d871 = SlotWidth"
equation "d872 = ( Depth ) - 2 * ( Wall + DeckClearance + RimBorder )"
equation "d873 = DeckThick"
equation "d875 = ( FootHeight ) + PanHeight - DeckThick"
equation "d877 = ( BaseX + LeftRun + FaucetGap ) + ( ( ( ( ( RightRun - ModuleGap ) / 2 ) - ( 10 * SlotPitch + SlotWidth ) ) / 2 ) + ( 6 * SlotPitch ) )"
equation "d878 = ( BaseY ) + ( Wall + DeckClearance + RimBorder )"
equation "d879 = SlotWidth"
equation "d880 = ( Depth ) - 2 * ( Wall + DeckClearance + RimBorder )"
equation "d881 = DeckThick"
equation "d883 = ( FootHeight ) + PanHeight - DeckThick"
equation "d885 = ( BaseX + LeftRun + FaucetGap ) + ( ( ( ( ( RightRun - ModuleGap ) / 2 ) - ( 10 * SlotPitch + SlotWidth ) ) / 2 ) + ( 7 * SlotPitch ) )"
equation "d886 = ( BaseY ) + ( Wall + DeckClearance + RimBorder )"
equation "d887 = SlotWidth"
equation "d888 = ( Depth ) - 2 * ( Wall + DeckClearance + RimBorder )"
equation "d889 = DeckThick"
equation "d891 = ( FootHeight ) + PanHeight - DeckThick"
equation "d893 = ( BaseX + LeftRun + FaucetGap ) + ( ( ( ( ( RightRun - ModuleGap ) / 2 ) - ( 10 * SlotPitch + SlotWidth ) ) / 2 ) + ( 8 * SlotPitch ) )"
equation "d894 = ( BaseY ) + ( Wall + DeckClearance + RimBorder )"
equation "d895 = SlotWidth"
equation "d896 = ( Depth ) - 2 * ( Wall + DeckClearance + RimBorder )"
equation "d897 = DeckThick"
equation "d899 = ( FootHeight ) + PanHeight - DeckThick"
equation "d901 = ( BaseX + LeftRun + FaucetGap ) + ( ( ( ( ( RightRun - ModuleGap ) / 2 ) - ( 10 * SlotPitch + SlotWidth ) ) / 2 ) + ( 9 * SlotPitch ) )"
equation "d902 = ( BaseY ) + ( Wall + DeckClearance + RimBorder )"
equation "d903 = SlotWidth"
equation "d904 = ( Depth ) - 2 * ( Wall + DeckClearance + RimBorder )"
equation "d905 = DeckThick"
equation "d907 = ( FootHeight ) + PanHeight - DeckThick"
equation "d909 = ( BaseX + LeftRun + FaucetGap ) + ( ( ( ( ( RightRun - ModuleGap ) / 2 ) - ( 10 * SlotPitch + SlotWidth ) ) / 2 ) + ( 10 * SlotPitch ) )"
equation "d910 = ( BaseY ) + ( Wall + DeckClearance + RimBorder )"
equation "d911 = SlotWidth"
equation "d912 = ( Depth ) - 2 * ( Wall + DeckClearance + RimBorder )"
equation "d913 = DeckThick"
equation "d915 = ( FootHeight ) + PanHeight - DeckThick"
equation "d917 = ( BaseX + LeftRun + FaucetGap ) + ( ( ( RightRun - ModuleGap ) / 2 ) / 2 - 8 mm )"
equation "d918 = ( BaseY ) + ( ( Depth ) - Wall - DeckClearance - 4 mm )"
equation "d921 = DeckThick"
equation "d925 = ( BaseX + LeftRun + FaucetGap ) + ( ( 11 mm ) - FootSize / 2 )"
equation "d926 = ( BaseY ) + ( ( 11 mm ) - FootSize / 2 )"
equation "d927 = FootSize"
equation "d928 = FootSize"
equation "d929 = FootHeight"
equation "d931 = FootHeight"
equation "d933 = ( BaseX + LeftRun + FaucetGap ) + ( ( 11 mm ) - PegSize / 2 )"
equation "d934 = ( BaseY ) + ( ( 11 mm ) - PegSize / 2 )"
equation "d935 = PegSize"
equation "d936 = PegSize"
equation "d937 = PegHeight"
equation "d941 = ( BaseX + LeftRun + FaucetGap ) + ( ( 11 mm ) - FootSize / 2 )"
equation "d942 = ( BaseY ) + ( ( ( Depth ) - 11 mm ) - FootSize / 2 )"
equation "d943 = FootSize"
equation "d944 = FootSize"
equation "d945 = FootHeight"
equation "d947 = FootHeight"
equation "d949 = ( BaseX + LeftRun + FaucetGap ) + ( ( 11 mm ) - PegSize / 2 )"
equation "d950 = ( BaseY ) + ( ( ( Depth ) - 11 mm ) - PegSize / 2 )"
equation "d951 = PegSize"
equation "d952 = PegSize"
equation "d953 = PegHeight"
equation "d957 = ( BaseX + LeftRun + FaucetGap ) + ( ( ( ( RightRun - ModuleGap ) / 2 ) - 11 mm ) - FootSize / 2 )"
equation "d958 = ( BaseY ) + ( ( 11 mm ) - FootSize / 2 )"
equation "d959 = FootSize"
equation "d960 = FootSize"
equation "d961 = FootHeight"
equation "d963 = FootHeight"
equation "d965 = ( BaseX + LeftRun + FaucetGap ) + ( ( ( ( RightRun - ModuleGap ) / 2 ) - 11 mm ) - PegSize / 2 )"
equation "d966 = ( BaseY ) + ( ( 11 mm ) - PegSize / 2 )"
equation "d967 = PegSize"
equation "d968 = PegSize"
equation "d969 = PegHeight"
equation "d973 = ( BaseX + LeftRun + FaucetGap ) + ( ( ( ( RightRun - ModuleGap ) / 2 ) - 11 mm ) - FootSize / 2 )"
equation "d974 = ( BaseY ) + ( ( ( Depth ) - 11 mm ) - FootSize / 2 )"
equation "d975 = FootSize"
equation "d976 = FootSize"
equation "d977 = FootHeight"
equation "d979 = FootHeight"
equation "d981 = ( BaseX + LeftRun + FaucetGap ) + ( ( ( ( RightRun - ModuleGap ) / 2 ) - 11 mm ) - PegSize / 2 )"
equation "d982 = ( BaseY ) + ( ( ( Depth ) - 11 mm ) - PegSize / 2 )"
equation "d983 = PegSize"
equation "d984 = PegSize"
equation "d985 = PegHeight"
equation "d987 = FootHeight"
equation "d989 = ( BaseX + LeftRun + FaucetGap + ( RightRun + ModuleGap ) / 2 ) + ( 0 mm )"
equation "d990 = ( BaseY ) + ( 0 mm )"
equation "d991 = ( RightRun - ModuleGap ) / 2"
equation "d992 = Depth"
equation "d993 = PanHeight"
equation "d997 = ( BaseX + LeftRun + FaucetGap + ( RightRun + ModuleGap ) / 2 ) + ( Wall )"
equation "d999 = -( -( ( FootHeight ) + FloorMin + DrainExtension * tan(DrainSlope) + ( ( Depth ) - ( Wall ) ) * tan(DrainSlope) ) )"
equation "d1000 = ( ( BaseY ) + ( Wall ) )"
equation "d1001 = -( -( ( FootHeight ) + FloorMin + DrainExtension * tan(DrainSlope) + ( ( Depth ) - ( ( Depth ) - Wall ) ) * tan(DrainSlope) ) )"
equation "d1002 = ( ( BaseY ) + ( ( Depth ) - Wall ) )"
equation "d1003 = -( -( ( FootHeight ) + PanHeight + 1 mm ) )"
equation "d1004 = ( ( RightRun - ModuleGap ) / 2 ) - 2 * Wall"
equation "d1006 = ( BaseX + LeftRun + FaucetGap + ( RightRun + ModuleGap ) / 2 ) + ( ( 18 mm ) - DrainWidth / 2 - Wall )"
equation "d1008 = -( -( FootHeight ) )"
equation "d1009 = ( ( BaseY ) + ( ( Depth ) - Wall ) )"
equation "d1010 = ( ( BaseY ) + ( ( Depth ) + DrainExtension ) )"
equation "d1011 = -( -( ( FootHeight ) + FloorMin + DrainExtension * tan(DrainSlope) + ( ( Depth ) - ( ( Depth ) + DrainExtension ) ) * tan(DrainSlope) ) )"
equation "d1012 = -( -( ( FootHeight ) + FloorMin + DrainExtension * tan(DrainSlope) + ( ( Depth ) - ( ( Depth ) - Wall ) ) * tan(DrainSlope) ) )"
equation "d1013 = DrainWidth + 2 * Wall"
equation "d1015 = ( BaseX + LeftRun + FaucetGap + ( RightRun + ModuleGap ) / 2 ) + ( ( 18 mm ) - DrainWidth / 2 - Wall )"
equation "d1017 = -( -( FootHeight ) )"
equation "d1018 = ( ( BaseY ) + ( ( Depth ) - Wall ) )"
equation "d1019 = ( ( BaseY ) + ( ( Depth ) + DrainExtension ) )"
equation "d1020 = -( -( ( ( FootHeight ) + FloorMin + DrainExtension * tan(DrainSlope) + ( ( Depth ) - ( ( Depth ) + DrainExtension ) ) * tan(DrainSlope) ) + ( 6 mm ) ) )"
equation "d1021 = -( -( ( ( FootHeight ) + FloorMin + DrainExtension * tan(DrainSlope) + ( ( Depth ) - ( ( Depth ) - Wall ) ) * tan(DrainSlope) ) + ( 6 mm ) ) )"
equation "d1022 = Wall"
equation "d1024 = ( BaseX + LeftRun + FaucetGap + ( RightRun + ModuleGap ) / 2 ) + ( ( 18 mm ) + DrainWidth / 2 )"
equation "d1026 = -( -( FootHeight ) )"
equation "d1027 = ( ( BaseY ) + ( ( Depth ) - Wall ) )"
equation "d1028 = ( ( BaseY ) + ( ( Depth ) + DrainExtension ) )"
equation "d1029 = -( -( ( ( FootHeight ) + FloorMin + DrainExtension * tan(DrainSlope) + ( ( Depth ) - ( ( Depth ) + DrainExtension ) ) * tan(DrainSlope) ) + ( 6 mm ) ) )"
equation "d1030 = -( -( ( ( FootHeight ) + FloorMin + DrainExtension * tan(DrainSlope) + ( ( Depth ) - ( ( Depth ) - Wall ) ) * tan(DrainSlope) ) + ( 6 mm ) ) )"
equation "d1031 = Wall"
equation "d1033 = ( BaseX + LeftRun + FaucetGap + ( RightRun + ModuleGap ) / 2 ) + ( ( 18 mm ) - DrainWidth / 2 )"
equation "d1035 = -( -( ( FootHeight ) + FloorMin + DrainExtension * tan(DrainSlope) + ( ( Depth ) - ( ( Depth ) - Wall ) ) * tan(DrainSlope) ) )"
equation "d1036 = ( ( BaseY ) + ( ( Depth ) - Wall ) )"
equation "d1037 = -( -( ( FootHeight ) + FloorMin + DrainExtension * tan(DrainSlope) + ( ( Depth ) - ( ( Depth ) + DrainExtension ) ) * tan(DrainSlope) ) )"
equation "d1038 = ( ( BaseY ) + ( ( Depth ) + DrainExtension ) )"
equation "d1039 = -( -( ( FootHeight ) + PanHeight + 1 mm ) )"
equation "d1040 = DrainWidth"
equation "d1042 = FootHeight"
equation "d1044 = ( BaseX + LeftRun + FaucetGap + ( RightRun + ModuleGap ) / 2 ) + ( Wall )"
equation "d1045 = ( BaseY ) + ( Wall )"
equation "d1048 = PanHeight - DeckThick"
equation "d1050 = FootHeight"
equation "d1052 = ( BaseX + LeftRun + FaucetGap + ( RightRun + ModuleGap ) / 2 ) + ( ( 18 mm ) + DrainWidth / 2 + 3 mm )"
equation "d1053 = ( BaseY ) + ( ( Depth ) - Wall - 12 mm )"
equation "d1056 = PanHeight - DeckThick"
equation "d1058 = FootHeight"
equation "d1060 = ( BaseX + LeftRun + FaucetGap + ( RightRun + ModuleGap ) / 2 ) + ( ( ( RightRun - ModuleGap ) / 2 ) - Wall - 12 mm )"
equation "d1061 = ( BaseY ) + ( Wall )"
equation "d1064 = PanHeight - DeckThick"
equation "d1066 = FootHeight"
equation "d1068 = ( BaseX + LeftRun + FaucetGap + ( RightRun + ModuleGap ) / 2 ) + ( ( ( RightRun - ModuleGap ) / 2 ) - Wall - 12 mm )"
equation "d1069 = ( BaseY ) + ( ( Depth ) - Wall - 12 mm )"
equation "d1072 = PanHeight - DeckThick"
equation "d1074 = ( BaseX + LeftRun + FaucetGap + ( RightRun + ModuleGap ) / 2 ) + ( ( 18 mm ) - DrainWidth / 2 - Wall )"
equation "d1076 = -( -( ( FootHeight ) - ( 0.2 mm ) ) )"
equation "d1077 = ( ( BaseY ) + ( ( Depth ) + DrainExtension - 2 mm ) )"
equation "d1078 = ( ( BaseY ) + ( ( ( Depth ) + DrainExtension - 2 mm ) + ( 1 mm ) ) )"
equation "d1079 = -( -( ( FootHeight ) + ( 0.6 mm ) ) )"
equation "d1080 = DrainWidth + 2 * Wall"
equation "d1082 = FootHeight"
equation "d1084 = ( BaseX + LeftRun + FaucetGap + ( RightRun + ModuleGap ) / 2 ) + ( ( 11 mm ) - PegSize / 2 - FitClearance )"
equation "d1085 = ( BaseY ) + ( ( 11 mm ) - PegSize / 2 - FitClearance )"
equation "d1086 = PegSize + 2 * FitClearance"
equation "d1087 = PegSize + 2 * FitClearance"
equation "d1088 = PegHeight + 0.3 mm"
equation "d1090 = FootHeight"
equation "d1092 = ( BaseX + LeftRun + FaucetGap + ( RightRun + ModuleGap ) / 2 ) + ( ( 11 mm ) - PegSize / 2 - FitClearance )"
equation "d1093 = ( BaseY ) + ( ( ( Depth ) - 11 mm ) - PegSize / 2 - FitClearance )"
equation "d1094 = PegSize + 2 * FitClearance"
equation "d1095 = PegSize + 2 * FitClearance"
equation "d1096 = PegHeight + 0.3 mm"
equation "d1098 = FootHeight"
equation "d1100 = ( BaseX + LeftRun + FaucetGap + ( RightRun + ModuleGap ) / 2 ) + ( ( ( ( RightRun - ModuleGap ) / 2 ) - 11 mm ) - PegSize / 2 - FitClearance )"
equation "d1101 = ( BaseY ) + ( ( 11 mm ) - PegSize / 2 - FitClearance )"
equation "d1102 = PegSize + 2 * FitClearance"
equation "d1103 = PegSize + 2 * FitClearance"
equation "d1104 = PegHeight + 0.3 mm"
equation "d1106 = FootHeight"
equation "d1108 = ( BaseX + LeftRun + FaucetGap + ( RightRun + ModuleGap ) / 2 ) + ( ( ( ( RightRun - ModuleGap ) / 2 ) - 11 mm ) - PegSize / 2 - FitClearance )"
equation "d1109 = ( BaseY ) + ( ( ( Depth ) - 11 mm ) - PegSize / 2 - FitClearance )"
equation "d1110 = PegSize + 2 * FitClearance"
equation "d1111 = PegSize + 2 * FitClearance"
equation "d1112 = PegHeight + 0.3 mm"
equation "d1114 = ( FootHeight ) + PanHeight - DeckThick"
equation "d1116 = ( BaseX + LeftRun + FaucetGap + ( RightRun + ModuleGap ) / 2 ) + ( Wall + DeckClearance )"
equation "d1117 = ( BaseY ) + ( Wall + DeckClearance )"
equation "d1118 = ( ( RightRun - ModuleGap ) / 2 ) - 2 * ( Wall + DeckClearance )"
equation "d1119 = ( Depth ) - 2 * ( Wall + DeckClearance )"
equation "d1120 = DeckThick"
equation "d1122 = ( FootHeight ) + PanHeight - DeckThick"
equation "d1124 = ( BaseX + LeftRun + FaucetGap + ( RightRun + ModuleGap ) / 2 ) + ( ( ( ( ( RightRun - ModuleGap ) / 2 ) - ( 10 * SlotPitch + SlotWidth ) ) / 2 ) + ( 0 * SlotPitch ) )"
equation "d1125 = ( BaseY ) + ( Wall + DeckClearance + RimBorder )"
equation "d1126 = SlotWidth"
equation "d1127 = ( Depth ) - 2 * ( Wall + DeckClearance + RimBorder )"
equation "d1128 = DeckThick"
equation "d1130 = ( FootHeight ) + PanHeight - DeckThick"
equation "d1132 = ( BaseX + LeftRun + FaucetGap + ( RightRun + ModuleGap ) / 2 ) + ( ( ( ( ( RightRun - ModuleGap ) / 2 ) - ( 10 * SlotPitch + SlotWidth ) ) / 2 ) + ( 1 * SlotPitch ) )"
equation "d1133 = ( BaseY ) + ( Wall + DeckClearance + RimBorder )"
equation "d1134 = SlotWidth"
equation "d1135 = ( Depth ) - 2 * ( Wall + DeckClearance + RimBorder )"
equation "d1136 = DeckThick"
equation "d1138 = ( FootHeight ) + PanHeight - DeckThick"
equation "d1140 = ( BaseX + LeftRun + FaucetGap + ( RightRun + ModuleGap ) / 2 ) + ( ( ( ( ( RightRun - ModuleGap ) / 2 ) - ( 10 * SlotPitch + SlotWidth ) ) / 2 ) + ( 2 * SlotPitch ) )"
equation "d1141 = ( BaseY ) + ( Wall + DeckClearance + RimBorder )"
equation "d1142 = SlotWidth"
equation "d1143 = ( Depth ) - 2 * ( Wall + DeckClearance + RimBorder )"
equation "d1144 = DeckThick"
equation "d1146 = ( FootHeight ) + PanHeight - DeckThick"
equation "d1148 = ( BaseX + LeftRun + FaucetGap + ( RightRun + ModuleGap ) / 2 ) + ( ( ( ( ( RightRun - ModuleGap ) / 2 ) - ( 10 * SlotPitch + SlotWidth ) ) / 2 ) + ( 3 * SlotPitch ) )"
equation "d1149 = ( BaseY ) + ( Wall + DeckClearance + RimBorder )"
equation "d1150 = SlotWidth"
equation "d1151 = ( Depth ) - 2 * ( Wall + DeckClearance + RimBorder )"
equation "d1152 = DeckThick"
equation "d1154 = ( FootHeight ) + PanHeight - DeckThick"
equation "d1156 = ( BaseX + LeftRun + FaucetGap + ( RightRun + ModuleGap ) / 2 ) + ( ( ( ( ( RightRun - ModuleGap ) / 2 ) - ( 10 * SlotPitch + SlotWidth ) ) / 2 ) + ( 4 * SlotPitch ) )"
equation "d1157 = ( BaseY ) + ( Wall + DeckClearance + RimBorder )"
equation "d1158 = SlotWidth"
equation "d1159 = ( Depth ) - 2 * ( Wall + DeckClearance + RimBorder )"
equation "d1160 = DeckThick"
equation "d1162 = ( FootHeight ) + PanHeight - DeckThick"
equation "d1164 = ( BaseX + LeftRun + FaucetGap + ( RightRun + ModuleGap ) / 2 ) + ( ( ( ( ( RightRun - ModuleGap ) / 2 ) - ( 10 * SlotPitch + SlotWidth ) ) / 2 ) + ( 5 * SlotPitch ) )"
equation "d1165 = ( BaseY ) + ( Wall + DeckClearance + RimBorder )"
equation "d1166 = SlotWidth"
equation "d1167 = ( Depth ) - 2 * ( Wall + DeckClearance + RimBorder )"
equation "d1168 = DeckThick"
equation "d1170 = ( FootHeight ) + PanHeight - DeckThick"
equation "d1172 = ( BaseX + LeftRun + FaucetGap + ( RightRun + ModuleGap ) / 2 ) + ( ( ( ( ( RightRun - ModuleGap ) / 2 ) - ( 10 * SlotPitch + SlotWidth ) ) / 2 ) + ( 6 * SlotPitch ) )"
equation "d1173 = ( BaseY ) + ( Wall + DeckClearance + RimBorder )"
equation "d1174 = SlotWidth"
equation "d1175 = ( Depth ) - 2 * ( Wall + DeckClearance + RimBorder )"
equation "d1176 = DeckThick"
equation "d1178 = ( FootHeight ) + PanHeight - DeckThick"
equation "d1180 = ( BaseX + LeftRun + FaucetGap + ( RightRun + ModuleGap ) / 2 ) + ( ( ( ( ( RightRun - ModuleGap ) / 2 ) - ( 10 * SlotPitch + SlotWidth ) ) / 2 ) + ( 7 * SlotPitch ) )"
equation "d1181 = ( BaseY ) + ( Wall + DeckClearance + RimBorder )"
equation "d1182 = SlotWidth"
equation "d1183 = ( Depth ) - 2 * ( Wall + DeckClearance + RimBorder )"
equation "d1184 = DeckThick"
equation "d1186 = ( FootHeight ) + PanHeight - DeckThick"
equation "d1188 = ( BaseX + LeftRun + FaucetGap + ( RightRun + ModuleGap ) / 2 ) + ( ( ( ( ( RightRun - ModuleGap ) / 2 ) - ( 10 * SlotPitch + SlotWidth ) ) / 2 ) + ( 8 * SlotPitch ) )"
equation "d1189 = ( BaseY ) + ( Wall + DeckClearance + RimBorder )"
equation "d1190 = SlotWidth"
equation "d1191 = ( Depth ) - 2 * ( Wall + DeckClearance + RimBorder )"
equation "d1192 = DeckThick"
equation "d1194 = ( FootHeight ) + PanHeight - DeckThick"
equation "d1196 = ( BaseX + LeftRun + FaucetGap + ( RightRun + ModuleGap ) / 2 ) + ( ( ( ( ( RightRun - ModuleGap ) / 2 ) - ( 10 * SlotPitch + SlotWidth ) ) / 2 ) + ( 9 * SlotPitch ) )"
equation "d1197 = ( BaseY ) + ( Wall + DeckClearance + RimBorder )"
equation "d1198 = SlotWidth"
equation "d1199 = ( Depth ) - 2 * ( Wall + DeckClearance + RimBorder )"
equation "d1200 = DeckThick"
equation "d1202 = ( FootHeight ) + PanHeight - DeckThick"
equation "d1204 = ( BaseX + LeftRun + FaucetGap + ( RightRun + ModuleGap ) / 2 ) + ( ( ( ( ( RightRun - ModuleGap ) / 2 ) - ( 10 * SlotPitch + SlotWidth ) ) / 2 ) + ( 10 * SlotPitch ) )"
equation "d1205 = ( BaseY ) + ( Wall + DeckClearance + RimBorder )"
equation "d1206 = SlotWidth"
equation "d1207 = ( Depth ) - 2 * ( Wall + DeckClearance + RimBorder )"
equation "d1208 = DeckThick"
equation "d1210 = ( FootHeight ) + PanHeight - DeckThick"